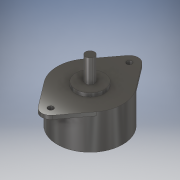
# Autodesk Inventor part: 14HM08
Saved by Autodesk Inventor 2019 (Build 230136000, 136)
## iProperties
Created: 2019-02-17
Part Number: 14HM08
Material: Generic
Document SubType Name: Modeling
Designer: Billy
Density: 1 g/cm^3
Appearance: Steel - Polished
Author: Billy
Autodesk Inventor part; units mm, degrees
ref_plane "YZ Plane" through (0, 0, 0) normal (1, 0, 0) x (0, 1, 0)
ref_plane "XZ Plane" through (0, 0, 0) normal (0, 1, 0) x (-1, 0, 0)
ref_plane "XY Plane" through (0, 0, 0) normal (0, 0, 1) x (1, 0, 0)
sketch "Sketch1" plane through (0, 0, 0) normal (0, 1, 0) x (-1, 0, 0)
  circle A0 centre (0, 0) radius 18.25
  dimension "d0" = 36.5
  constraints: 1 centre point, 1 coincident
  measures "d0" diameter of A0
extrude "Extrusion1" add sketch "Sketch1" along normal blind 19.5
sketch "Sketch2" plane through (0, 19.5, 0) normal (0, 1, 0) x (1, 0, 0)
  circle A0 centre (0, 0) radius 8
  dimension "d3" = 16
  constraints: 1 centre point, 1 coincident
  measures "d3" diameter of A0
extrude "Extrusion2" add sketch "Sketch2" along normal blind 2
sketch "Sketch3" plane through (0, 19.5, 0) normal (0, 1, 0) x (1, 0, 0)
  circle A0 centre (0, 21.95) radius 1.5
  circle A1 centre (0, -21.95) radius 1.5
  arc A2 (3.9863, 24.9682) -> (-3.9863, 24.9682) centre (0, 21.95) ccw
  circle A3 centre (0, 0) radius 8
  line L0 (-14.5499, -11.0165) -> (-3.9863, -24.9682)
  line L1 (-14.5499, 11.0165) -> (-3.9863, 24.9682)
  line L2 (14.5499, -11.0165) -> (3.9863, -24.9682)
  line L3 (14.5499, 11.0165) -> (3.9863, 24.9682)
  arc A4 (-14.5499, -11.0165) -> (14.5499, -11.0165) centre (0, 0) ccw
  arc A5 (3.0557, 17.9924) -> (-3.0557, 17.9924) centre (0, 0) ccw
  arc A6 (-3.9863, -24.9682) -> (3.9863, -24.9682) centre (0, -21.95) ccw
  arc A7 (3.0557, -17.9924) -> (-3.0557, -17.9924) centre (0, -21.95) ccw
  arc A8 (-14.5499, -11.0165) -> (14.5499, -11.0165) centre (0, 0) ccw
  arc A9 (14.5499, 11.0165) -> (-14.5499, 11.0165) centre (0, 0) ccw
  constraints: 18 point on circle, 10 centre point, 8 end point, 4 tangent, 2 coincident, 5 other
extrude "Extrusion3" add sketch "Sketch3" against normal blind 2 contours L3 A9 A5 L1 A2 | A4 L2 A6 L0
sketch "Sketch4" plane through (0, 21.5, 0) normal (0, 1, 0) x (1, 0, 0)
  circle A0 centre (0, 0) radius 2.5
  dimension "d12" = 5
  constraints: 1 centre point, 1 coincident
  measures "d12" diameter of A0
extrude "Extrusion4" add sketch "Sketch4" along normal blind 13
body "Solid1"
